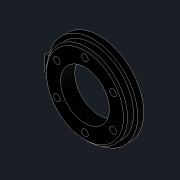
# Autodesk Inventor part: base11
Saved by Autodesk Inventor 2022 (Build 260153000, 153)
## iProperties
Created: 2021-07-30
Part Number: base11
Material: ABS プラスチック
Document SubType Name: Modeling
Designer: yuta0
Density: 1.06 g/cm^3
Appearance: 滑らか - 黒
Mass: 6.38316 g
Surface Area: 38.3222 cm^2
Volume: 6.02185 cm^3
購入先: 印刷
在庫数: 0.0
Author: yuta0
Autodesk Inventor part; units mm, degrees
ref_plane "YZ Plane" through (0, 0, 0) normal (1, 0, 0) x (0, 1, 0)
ref_plane "XZ Plane" through (0, 0, 0) normal (0, 1, 0) x (-1, 0, 0)
ref_plane "XY Plane" through (0, 0, 0) normal (0, 0, 1) x (1, 0, 0)
sketch "スケッチ1" plane through (0, 0, 0) normal (1, 0, 0) x (0, 1, 0)
  line L0 (12, 0) -> (12, -7)
  line L1 (22, -7) -> (22, -4)
  line L2 (22, -4) -> (20, -4)
  line L3 (20, -4) -> (20, 0)
  line L4 (20, 0) -> (12, 0)
  line L5 (0, -8.4) -> (0, 1.4) projected
  line L6 (22, -7) -> (12, -7)
  point P0 (0, 0)
  dimension "d0" = 20
  dimension "d1" = 2
  dimension "d2" = 4
  dimension "d3" = 3
  dimension "d4" = 8
  constraints: 12 end point, 5 perpendicular, 1 horizontal alignment, 1 vertical
  measures "d0" distance from line of point (0, 0) L3
  measures "d1" distance of L1.end L2.end
  measures "d2" distance of L2.end L3.end
  measures "d3" distance of L1.start L1.end
  measures "d4" distance of L3.end L0.start
revolve "回転1" add sketch "スケッチ1" angle 360 about axis through (0, 0, -10) along (0, 0, 1)
sketch "スケッチ2" plane through (0, 0, 0) normal (0, 0, 1) x (1, 0, 0)
  circle A0 centre (0, 0) radius 20 projected
  circle A1 centre (0, 0) radius 16
  point P0 (0, 16)
  point P1 (-13.8564, 8)
  point P2 (-13.8564, -8)
  point P3 (0, -16)
  point P4 (13.8564, -8)
  point P5 (13.8564, 8)
  dimension "d8" = 4
  dimension "d11" = 360
  constraints: 1 vertical alignment, 9 other
hole "穴1" at (0, 16, 0) at (-13.8564, 8, 0) at (-13.8564, -8, 0) at (0, -16, 0) at (13.8564, -8, 0) at (13.8564, 8, 0) direction (0, 0, -1) diameter 3.2 end through all clearance for "Socket Head Cap Screw" size "M3" standard "Ansi Metric M Profile"
chamfer "面取り1" distance 1 angle 45 1 edges at (0, -20, 0)
sketch "スケッチ3" plane through (0, 0, -7) normal (0, 0, -1) x (-1, 0, 0)
  circle A0 centre (0, 0) radius 22 projected
  circle A1 centre (0, 0) radius 24
  line L0 (0, 0) -> (23.6354, -4.1676)
  line L1 (0, 0) -> (23.6354, 4.1676)
  line L2 (-35, 0) -> (35, 0) projected
  point P0 (21.6658, -3.8203)
  point P1 (21.6658, 3.8203)
  dimension "d23" = 2
  dimension "d24" = 10
  dimension "d25" = 10
  constraints: 4 end point, 2 point on circle, 1 centre point, 1 coincident
  measures "d23" radial gap between concentric circles of A1 A0
  measures "d24" angle of L0 L2
  measures "d25" angle of L2 L1
extrude "押し出し1" add sketch "スケッチ3" against normal up to surface (3 mm away) contours L2 A1 L0 A0 | A0 L1 A1 L2 picked at (23.0463, -3.5914) picked at (23.1081, 3.1693)
fillet "フィレット1" radius 0.5 4 edges at (-23.6354, -4.1676, -5.5) (-21.6658, -3.8203, -5.5) (-23.6354, 4.1676, -5.5) (-21.6658, 3.8203, -5.5)
equation "\"d25\" = d24"
